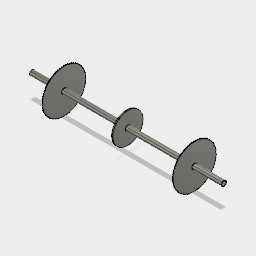
torsional analysis (Autodesk Fusion 360 design; units mm, degrees)
Autodesk Fusion 360 part; units mm, degrees
note: some values were not read from the file. Chosen so that the rebuilt part matches the saved one: which face or edge a step refers to; that a step has no effect.
sketch "Sketch1" plane through (0, 0, 0) normal (0, 0, 1) x (1, 0, 0)
  line L0 (0, 0) -> (-914.4, 0)
  dimension "d1" = 914.4
  measures "d1" distance of L0.start L0.end
pipe "Pipe1" add diameter 25.4 wall 2 path "Sketch1" along L0
ref_plane "WorkPlane1" through (-140, 0, 0) normal (1, 0, 0) x (0, 0, -1)
sketch "Sketch2" plane through (-140, 0, 0) normal (1, 0, 0) x (0, 0, -1)
  line L0 (-0.0125, 104.6) -> (0.9875, 104.6)
  line L1 (-0.0125, 104.6) -> (-1.0125, 104.6)
  line L2 (-9.8073, 104.1392) -> (-8.8117, 104.2329)
  line L3 (-9.8073, 104.1392) -> (-10.8029, 104.0456)
  line L4 (-19.516, 102.7633) -> (-18.5335, 102.9497)
  line L5 (-19.516, 102.7633) -> (-20.4984, 102.5768)
  line L6 (-29.0531, 100.4842) -> (-28.0924, 100.7619)
  line L7 (-29.0531, 100.4842) -> (-30.0138, 100.2066)
  line L8 (-38.3349, 97.3221) -> (-37.4045, 97.6885)
  line L9 (-38.3349, 97.3221) -> (-39.2654, 96.9557)
  line L10 (-47.2799, 93.3047) -> (-46.3878, 93.7566)
  line L11 (-47.2799, 93.3047) -> (-48.172, 92.8528)
  line L12 (-55.8093, 88.4674) -> (-54.9635, 89.0008)
  line L13 (-55.8093, 88.4674) -> (-56.6552, 87.9339)
  line L14 (-63.8483, 82.8526) -> (-63.0562, 83.4629)
  line L15 (-63.8483, 82.8526) -> (-64.6405, 82.2423)
  line L16 (-71.3262, 76.5097) -> (-70.5947, 77.1915)
  line L17 (-71.3262, 76.5097) -> (-72.0577, 75.8279)
  line L18 (-78.1773, 69.4944) -> (-77.5128, 70.2417)
  line L19 (-78.1773, 69.4944) -> (-78.8418, 68.7471)
  line L20 (-84.3413, 61.8684) -> (-83.7498, 62.6747)
  line L21 (-84.3413, 61.8684) -> (-84.9329, 61.0622)
  line L22 (-89.7642, 53.6987) -> (-89.2507, 54.5568)
  line L23 (-89.7642, 53.6987) -> (-90.2777, 52.8406)
  line L24 (-94.3982, 45.0571) -> (-93.9673, 45.9595)
  line L25 (-94.3982, 45.0571) -> (-94.829, 44.1547)
  line L26 (-98.2026, 36.0195) -> (-97.8581, 36.9583)
  line L27 (-98.2026, 36.0195) -> (-98.5471, 35.0807)
  line L28 (-101.144, 26.6654) -> (-100.889, 27.6324)
  line L29 (-101.144, 26.6654) -> (-101.3991, 25.6985)
  line L30 (-103.1966, 17.077) -> (-103.0332, 18.0635)
  line L31 (-103.1966, 17.077) -> (-103.36, 16.0904)
  line L32 (-104.3423, 7.3385) -> (-104.272, 8.336)
  line L33 (-104.3423, 7.3385) -> (-104.4125, 6.3409)
  line L34 (-104.571, -2.4645) -> (-104.5944, -1.4648)
  line L35 (-104.571, -2.4645) -> (-104.5475, -3.4643)
  line L36 (-103.8807, -12.2459) -> (-103.9976, -11.2528)
  line L37 (-103.8807, -12.2459) -> (-103.7637, -13.239)
  line L38 (-102.2775, -21.9196) -> (-102.487, -20.9418)
  line L39 (-102.2775, -21.9196) -> (-102.0681, -22.8975)
  line L40 (-99.7755, -31.4007) -> (-100.0756, -30.4468)
  line L41 (-99.7755, -31.4007) -> (-99.4754, -32.3546)
  line L42 (-96.3967, -40.6059) -> (-96.7848, -39.6843)
  line L43 (-96.3967, -40.6059) -> (-96.0086, -41.5275)
  line L44 (-92.1707, -49.4542) -> (-92.6434, -48.573)
  line L45 (-92.1707, -49.4542) -> (-91.698, -50.3354)
  line L46 (-87.1348, -57.8679) -> (-87.6879, -57.0348)
  line L47 (-87.1348, -57.8679) -> (-86.5816, -58.701)
  line L48 (-81.3331, -65.7731) -> (-81.9618, -64.9954)
  line L49 (-81.3331, -65.7731) -> (-80.7043, -66.5507)
  line L50 (-74.8166, -73.1002) -> (-75.5154, -72.3848)
  line L51 (-74.8166, -73.1002) -> (-74.1178, -73.8155)
  line L52 (-67.6426, -79.7849) -> (-68.4053, -79.1382)
  line L53 (-67.6426, -79.7849) -> (-66.8799, -80.4317)
  line L54 (-59.8742, -85.7685) -> (-60.6941, -85.196)
  line L55 (-59.8742, -85.7685) -> (-59.0543, -86.341)
  line L56 (-51.5797, -90.9983) -> (-52.4496, -90.5051)
  line L57 (-51.5797, -90.9983) -> (-50.7097, -91.4916)
  line L58 (-42.8318, -95.4285) -> (-43.7441, -95.0189)
  line L59 (-42.8318, -95.4285) -> (-41.9195, -95.8381)
  line L60 (-33.7075, -99.02) -> (-34.6541, -98.6976)
  line L61 (-33.7075, -99.02) -> (-32.7609, -99.3424)
  line L62 (-24.287, -101.7413) -> (-25.2597, -101.509)
  line L63 (-24.287, -101.7413) -> (-23.3144, -101.9736)
  line L64 (-14.6531, -103.5686) -> (-15.6432, -103.4284)
  line L65 (-14.6531, -103.5686) -> (-13.663, -103.7088)
  line L66 (-4.8904, -104.4856) -> (-5.8893, -104.4387)
  line L67 (-4.8904, -104.4856) -> (-3.8915, -104.5325)
  line L68 (4.9153, -104.4844) -> (3.9164, -104.5313)
  line L69 (4.9153, -104.4844) -> (5.9142, -104.4376)
  line L70 (14.6778, -103.5651) -> (13.6876, -103.7053)
  line L71 (14.6778, -103.5651) -> (15.6679, -103.4249)
  line L72 (24.3113, -101.7356) -> (23.3386, -101.9679)
  line L73 (24.3113, -101.7356) -> (25.2839, -101.5032)
  line L74 (33.7311, -99.012) -> (32.7845, -99.3343)
  line L75 (33.7311, -99.012) -> (34.6777, -98.6896)
  line L76 (42.8545, -95.4183) -> (41.9422, -95.8279)
  line L77 (42.8545, -95.4183) -> (43.7668, -95.0087)
  line L78 (51.6013, -90.9861) -> (50.7314, -91.4793)
  line L79 (51.6013, -90.9861) -> (52.4712, -90.4928)
  line L80 (59.8947, -85.7542) -> (59.0748, -86.3268)
  line L81 (59.8947, -85.7542) -> (60.7146, -85.1817)
  line L82 (67.6616, -79.7688) -> (66.8989, -80.4156)
  line L83 (67.6616, -79.7688) -> (68.4243, -79.122)
  line L84 (74.834, -73.0824) -> (74.1352, -73.7977)
  line L85 (74.834, -73.0824) -> (75.5328, -72.367)
  line L86 (81.3487, -65.7537) -> (80.72, -66.5313)
  line L87 (81.3487, -65.7537) -> (81.9774, -64.976)
  line L88 (87.1485, -57.8471) -> (86.5954, -58.6802)
  line L89 (87.1485, -57.8471) -> (87.7017, -57.014)
  line L90 (92.1825, -49.4322) -> (91.7098, -50.3135)
  line L91 (92.1825, -49.4322) -> (92.6552, -48.551)
  line L92 (96.4064, -40.5829) -> (96.0183, -41.5045)
  line L93 (96.4064, -40.5829) -> (96.7944, -39.6613)
  line L94 (99.783, -31.377) -> (99.4829, -32.3309)
  line L95 (99.783, -31.377) -> (100.0831, -30.4231)
  line L96 (102.2827, -21.8953) -> (102.0733, -22.8731)
  line L97 (102.2827, -21.8953) -> (102.4922, -20.9175)
  line L98 (103.8836, -12.2212) -> (103.7666, -13.2143)
  line L99 (103.8836, -12.2212) -> (104.0006, -11.228)
  line L100 (104.5715, -2.4396) -> (104.5481, -3.4394)
  line L101 (104.5715, -2.4396) -> (104.595, -1.4399)
  line L102 (104.3405, 7.3633) -> (104.4108, 6.3658)
  line L103 (104.3405, 7.3633) -> (104.2702, 8.3608)
  line L104 (103.1925, 17.1016) -> (103.3559, 16.115)
  line L105 (103.1925, 17.1016) -> (103.0291, 18.0881)
  line L106 (101.1377, 26.6895) -> (101.3927, 25.7226)
  line L107 (101.1377, 26.6895) -> (100.8826, 27.6564)
  line L108 (98.194, 36.0429) -> (98.5385, 35.1041)
  line L109 (98.194, 36.0429) -> (97.8496, 36.9817)
  line L110 (94.3875, 45.0796) -> (94.8183, 44.1772)
  line L111 (94.3875, 45.0796) -> (93.9566, 45.982)
  line L112 (89.7514, 53.7201) -> (90.2649, 52.862)
  line L113 (89.7514, 53.7201) -> (89.2379, 54.5782)
  line L114 (84.3266, 61.8885) -> (84.9182, 61.0822)
  line L115 (84.3266, 61.8885) -> (83.735, 62.6947)
  line L116 (78.1607, 69.513) -> (78.8252, 68.7657)
  line L117 (78.1607, 69.513) -> (77.4963, 70.2603)
  line L118 (71.308, 76.5267) -> (72.0395, 75.8449)
  line L119 (71.308, 76.5267) -> (70.5765, 77.2085)
  line L120 (63.8286, 82.8678) -> (64.6207, 82.2575)
  line L121 (63.8286, 82.8678) -> (63.0364, 83.4781)
  line L122 (55.7883, 88.4807) -> (56.6341, 87.9472)
  line L123 (55.7883, 88.4807) -> (54.9424, 89.0141)
  line L124 (47.2577, 93.316) -> (48.1497, 92.8641)
  line L125 (47.2577, 93.316) -> (46.3656, 93.7679)
  line L126 (38.3118, 97.3312) -> (39.2422, 96.9649)
  line L127 (38.3118, 97.3312) -> (37.3813, 97.6976)
  line L128 (29.0292, 100.4911) -> (29.9899, 100.2135)
  line L129 (29.0292, 100.4911) -> (28.0685, 100.7688)
  line L130 (19.4915, 102.7679) -> (20.4739, 102.5814)
  line L131 (19.4915, 102.7679) -> (18.509, 102.9544)
  line L132 (9.7825, 104.1416) -> (10.7781, 104.0479)
  line L133 (9.7825, 104.1416) -> (8.7869, 104.2352)
  arc A0 (0.9875, 104.6) -> (8.7869, 104.2352) centre (4.9379, 105.5011) ccw
  arc A1 (-8.8117, 104.2329) -> (-1.0125, 104.6) centre (-4.9631, 105.4999) ccw
  arc A2 (-18.5335, 102.9497) -> (-10.8029, 104.0456) centre (-14.8204, 104.5716) ccw
  arc A3 (-28.0924, 100.7619) -> (-20.4984, 102.5768) centre (-24.5476, 102.7243) ccw
  arc A4 (-37.4045, 97.6885) -> (-30.0138, 100.2066) centre (-34.0589, 99.9742) ccw
  arc A5 (-46.3878, 93.7566) -> (-39.2654, 96.9557) centre (-43.271, 96.3456) ccw
  arc A6 (-54.9635, 89.0008) -> (-48.172, 92.8528) centre (-52.1028, 91.8703) ccw
  arc A7 (-63.0562, 83.4629) -> (-56.6552, 87.9339) centre (-60.4768, 86.5876) ccw
  arc A8 (-70.5947, 77.1915) -> (-64.6405, 82.2423) centre (-68.3192, 80.544) ccw
  arc A9 (-77.5128, 70.2417) -> (-72.0577, 75.8279) centre (-75.5613, 73.7926) ccw
  arc A10 (-83.7498, 62.6747) -> (-78.8418, 68.7471) centre (-82.1393, 66.3927) ccw
  arc A11 (-89.2507, 54.5568) -> (-84.9329, 61.0622) centre (-87.9955, 58.4093) ccw
  arc A12 (-93.9673, 45.9595) -> (-90.2777, 52.8406) centre (-93.0784, 49.9126) ccw
  arc A13 (-97.8581, 36.9583) -> (-94.829, 44.1547) centre (-97.3433, 40.9773) ccw
  arc A14 (-100.889, 27.6324) -> (-98.5471, 35.0807) centre (-100.7528, 31.6819) ccw
  arc A15 (-103.0332, 18.0635) -> (-101.3991, 25.6985) centre (-103.2768, 22.108) ccw
  arc A16 (-104.272, 8.336) -> (-103.36, 16.0904) centre (-104.8932, 12.3399) ccw
  arc A17 (-104.5944, -1.4648) -> (-104.4125, 6.3409) centre (-105.5878, 2.4633) ccw
  arc A18 (-103.9976, -11.2528) -> (-104.5475, -3.4643) centre (-105.3546, -7.4349) ccw
  arc A19 (-102.487, -20.9418) -> (-103.7637, -13.239) centre (-104.1954, -17.2678) ccw
  arc A20 (-100.0756, -30.4468) -> (-102.0681, -22.8975) centre (-102.1206, -26.9489) ccw
  arc A21 (-96.7848, -39.6843) -> (-99.4754, -32.3546) centre (-99.1483, -36.3932) ccw
  arc A22 (-92.6434, -48.573) -> (-96.0086, -41.5275) centre (-95.3048, -45.5177) ccw
  arc A23 (-87.6879, -57.0348) -> (-91.698, -50.3354) centre (-90.6236, -54.2422) ccw
  arc A24 (-81.9618, -64.9954) -> (-86.5816, -58.701) centre (-85.1461, -62.49) ccw
  arc A25 (-75.5154, -72.3848) -> (-80.7043, -66.5507) centre (-78.9203, -70.1886) ccw
  arc A26 (-68.4053, -79.1382) -> (-74.1178, -73.8155) centre (-72.001, -77.2704) ccw
  arc A27 (-60.6941, -85.196) -> (-66.8799, -80.4317) centre (-64.4489, -83.6732) ccw
  arc A28 (-52.4496, -90.5051) -> (-59.0543, -86.341) centre (-56.3304, -89.3406) ccw
  arc A29 (-43.7441, -95.0189) -> (-50.7097, -91.4916) centre (-47.7169, -94.2229) ccw
  arc A30 (-34.6541, -98.6976) -> (-41.9195, -95.8381) centre (-38.6841, -98.2772) ccw
  arc A31 (-25.2597, -101.509) -> (-32.7609, -99.3424) centre (-29.3113, -101.4678) ccw
  arc A32 (-15.6432, -103.4284) -> (-23.3144, -101.9736) centre (-19.6809, -103.7667) ccw
  arc A33 (-5.8893, -104.4387) -> (-13.663, -103.7088) centre (-9.8775, -105.1537) ccw
  arc A34 (3.9164, -104.5313) -> (-3.8915, -104.5325) centre (0.0126, -105.6166) ccw
  arc A35 (13.6876, -103.7053) -> (5.9142, -104.4376) centre (9.9026, -105.1513) ccw
  arc A36 (23.3386, -101.9679) -> (15.6679, -103.4249) centre (19.7057, -103.762) ccw
  arc A37 (32.7845, -99.3343) -> (25.2839, -101.5032) centre (29.3355, -101.4608) ccw
  arc A38 (41.9422, -95.8279) -> (34.6777, -98.6896) centre (38.7075, -98.2679) ccw
  arc A39 (50.7314, -91.4793) -> (43.7668, -95.0087) centre (47.7394, -94.2115) ccw
  arc A40 (59.0748, -86.3268) -> (52.4712, -90.4928) centre (56.3517, -89.3272) ccw
  arc A41 (66.8989, -80.4156) -> (60.7146, -85.1817) centre (64.4689, -83.6578) ccw
  arc A42 (74.1352, -73.7977) -> (68.4243, -79.122) centre (72.0194, -77.2532) ccw
  arc A43 (80.72, -66.5313) -> (75.5328, -72.367) centre (78.9371, -70.1698) ccw
  arc A44 (86.5954, -58.6802) -> (81.9774, -64.976) centre (85.161, -62.4697) ccw
  arc A45 (91.7098, -50.3135) -> (87.7017, -57.014) centre (90.6366, -54.2206) ccw
  arc A46 (96.0183, -41.5045) -> (92.6552, -48.551) centre (95.3156, -45.495) ccw
  arc A47 (99.4829, -32.3309) -> (96.7944, -39.6613) centre (99.157, -36.3696) ccw
  arc A48 (102.0733, -22.8731) -> (100.0831, -30.4231) centre (102.127, -26.9246) ccw
  arc A49 (103.7666, -13.2143) -> (102.4922, -20.9175) centre (104.1995, -17.2429) ccw
  arc A50 (104.5481, -3.4394) -> (104.0006, -11.228) centre (105.3563, -7.4098) ccw
  arc A51 (104.4108, 6.3658) -> (104.595, -1.4399) centre (105.5872, 2.4885) ccw
  arc A52 (103.3559, 16.115) -> (104.2702, 8.3608) centre (104.8903, 12.3649) ccw
  arc A53 (101.3927, 25.7226) -> (103.0291, 18.0881) centre (103.2715, 22.1327) ccw
  arc A54 (98.5385, 35.1041) -> (100.8826, 27.6564) centre (100.7452, 31.7059) ccw
  arc A55 (94.8183, 44.1772) -> (97.8496, 36.9817) centre (97.3335, 41.0005) ccw
  arc A56 (90.2649, 52.862) -> (93.9566, 45.982) centre (93.0665, 49.9348) ccw
  arc A57 (84.9182, 61.0822) -> (89.2379, 54.5782) centre (87.9816, 58.4303) ccw
  arc A58 (78.8252, 68.7657) -> (83.735, 62.6947) centre (82.1235, 66.4123) ccw
  arc A59 (72.0395, 75.8449) -> (77.4963, 70.2603) centre (75.5437, 73.8106) ccw
  arc A60 (64.6207, 82.2575) -> (70.5765, 77.2085) centre (68.3, 80.5603) ccw
  arc A61 (56.6341, 87.9472) -> (63.0364, 83.4781) centre (60.4561, 86.6021) ccw
  arc A62 (48.1497, 92.8641) -> (54.9424, 89.0141) centre (52.0809, 91.8827) ccw
  arc A63 (39.2422, 96.9649) -> (46.3656, 93.7679) centre (43.248, 96.3559) ccw
  arc A64 (29.9899, 100.2135) -> (37.3813, 97.6976) centre (34.0351, 99.9824) ccw
  arc A65 (20.4739, 102.5814) -> (28.0685, 100.7688) centre (24.523, 102.7301) ccw
  arc A66 (10.7781, 104.0479) -> (18.509, 102.9544) centre (14.7955, 104.5751) ccw
  dimension "d9" = 1
  dimension "d10" = 1
  dimension "d12" = 360
  dimension "d14" = 360
  measures "d9" distance of L0.start L0.end
  measures "d10" distance of L0.start L1.end
ref_plane "WorkPlane3" through (-764.4, 0, 0) normal (-1, 0, 0) x (0, 0, 1)
sketch "Sketch3" plane through (-764.4, 0, 0) normal (-1, 0, 0) x (0, 0, -1)
  line L0 (-0.0279, -104.6) -> (0.9721, -104.6)
  line L1 (-0.0279, -104.6) -> (-1.0279, -104.6)
  line L2 (9.7672, -104.143) -> (8.7716, -104.2366)
  line L3 (9.7672, -104.143) -> (10.7628, -104.0494)
  line L4 (19.4764, -102.7708) -> (18.4939, -102.9572)
  line L5 (19.4764, -102.7708) -> (20.4588, -102.5843)
  line L6 (29.0144, -100.4954) -> (28.0537, -100.773)
  line L7 (29.0144, -100.4954) -> (29.9751, -100.2178)
  line L8 (38.2974, -97.3369) -> (37.367, -97.7033)
  line L9 (38.2974, -97.3369) -> (39.2279, -96.9705)
  line L10 (47.2439, -93.3229) -> (46.3519, -93.7748)
  line L11 (47.2439, -93.3229) -> (48.136, -92.871)
  line L12 (55.7752, -88.4889) -> (54.9294, -89.0223)
  line L13 (55.7752, -88.4889) -> (56.6211, -87.9554)
  line L14 (63.8164, -82.8772) -> (63.0242, -83.4875)
  line L15 (63.8164, -82.8772) -> (64.6086, -82.2669)
  line L16 (71.2967, -76.5372) -> (70.5652, -77.219)
  line L17 (71.2967, -76.5372) -> (72.0283, -75.8554)
  line L18 (78.1505, -69.5245) -> (77.486, -70.2718)
  line L19 (78.1505, -69.5245) -> (78.815, -68.7772)
  line L20 (84.3175, -61.9009) -> (83.7259, -62.7072)
  line L21 (84.3175, -61.9009) -> (84.9091, -61.0947)
  line L22 (89.7435, -53.7333) -> (89.23, -54.5914)
  line L23 (89.7435, -53.7333) -> (90.257, -52.8752)
  line L24 (94.3808, -45.0935) -> (93.95, -45.9959)
  line L25 (94.3808, -45.0935) -> (94.8117, -44.1911)
  line L26 (98.1887, -36.0574) -> (97.8443, -36.9962)
  line L27 (98.1887, -36.0574) -> (98.5332, -35.1186)
  line L28 (101.1337, -26.7044) -> (100.8787, -27.6713)
  line L29 (101.1337, -26.7044) -> (101.3888, -25.7375)
  line L30 (103.19, -17.1168) -> (103.0266, -18.1033)
  line L31 (103.19, -17.1168) -> (103.3534, -16.1302)
  line L32 (104.3394, -7.3787) -> (104.2691, -8.3762)
  line L33 (104.3394, -7.3787) -> (104.4097, -6.3811)
  line L34 (104.5719, 2.4242) -> (104.5953, 1.4245)
  line L35 (104.5719, 2.4242) -> (104.5485, 3.424)
  line L36 (103.8854, 12.2059) -> (104.0024, 11.2127)
  line L37 (103.8854, 12.2059) -> (103.7684, 13.199)
  line L38 (102.286, 21.8802) -> (102.4954, 20.9024)
  line L39 (102.286, 21.8802) -> (102.0765, 22.858)
  line L40 (99.7876, 31.3623) -> (100.0877, 30.4084)
  line L41 (99.7876, 31.3623) -> (99.4875, 32.3162)
  line L42 (96.4123, 40.5687) -> (96.8004, 39.6471)
  line L43 (96.4123, 40.5687) -> (96.0242, 41.4904)
  line L44 (92.1898, 49.4187) -> (92.6625, 48.5374)
  line L45 (92.1898, 49.4187) -> (91.7171, 50.2999)
  line L46 (87.1571, 57.8343) -> (87.7102, 57.0012)
  line L47 (87.1571, 57.8343) -> (86.6039, 58.6674)
  line L48 (81.3584, 65.7417) -> (81.9871, 64.9641)
  line L49 (81.3584, 65.7417) -> (80.7297, 66.5193)
  line L50 (74.8448, 73.0714) -> (75.5435, 72.356)
  line L51 (74.8448, 73.0714) -> (74.146, 73.7867)
  line L52 (67.6734, 79.7589) -> (68.4361, 79.1121)
  line L53 (67.6734, 79.7589) -> (66.9107, 80.4056)
  line L54 (59.9073, 85.7454) -> (60.7272, 85.1729)
  line L55 (59.9073, 85.7454) -> (59.0874, 86.3179)
  line L56 (51.6147, 90.9785) -> (52.4846, 90.4852)
  line L57 (51.6147, 90.9785) -> (50.7448, 91.4717)
  line L58 (42.8686, 95.412) -> (43.7808, 95.0024)
  line L59 (42.8686, 95.412) -> (41.9563, 95.8216)
  line L60 (33.7457, 99.007) -> (34.6923, 98.6847)
  line L61 (33.7457, 99.007) -> (32.7991, 99.3294)
  line L62 (24.3262, 101.732) -> (25.2989, 101.4997)
  line L63 (24.3262, 101.732) -> (23.3536, 101.9643)
  line L64 (14.693, 103.5629) -> (15.6831, 103.4227)
  line L65 (14.693, 103.5629) -> (13.7029, 103.7031)
  line L66 (4.9307, 104.4837) -> (5.9296, 104.4369)
  line L67 (4.9307, 104.4837) -> (3.9318, 104.5306)
  line L68 (-4.875, 104.4863) -> (-3.8761, 104.5332)
  line L69 (-4.875, 104.4863) -> (-5.8739, 104.4395)
  line L70 (-14.6379, 103.5707) -> (-13.6477, 103.7109)
  line L71 (-14.6379, 103.5707) -> (-15.628, 103.4305)
  line L72 (-24.272, 101.7449) -> (-23.2994, 101.9772)
  line L73 (-24.272, 101.7449) -> (-25.2447, 101.5126)
  line L74 (-33.6929, 99.025) -> (-32.7463, 99.3473)
  line L75 (-33.6929, 99.025) -> (-34.6396, 98.7026)
  line L76 (-42.8177, 95.4348) -> (-41.9055, 95.8444)
  line L77 (-42.8177, 95.4348) -> (-43.73, 95.0252)
  line L78 (-51.5663, 91.0059) -> (-50.6963, 91.4992)
  line L79 (-51.5663, 91.0059) -> (-52.4362, 90.5127)
  line L80 (-59.8616, 85.7773) -> (-59.0417, 86.3498)
  line L81 (-59.8616, 85.7773) -> (-60.6815, 85.2048)
  line L82 (-67.6309, 79.7949) -> (-66.8682, 80.4417)
  line L83 (-67.6309, 79.7949) -> (-68.3936, 79.1481)
  line L84 (-74.8058, 73.1112) -> (-74.1071, 73.8266)
  line L85 (-74.8058, 73.1112) -> (-75.5046, 72.3959)
  line L86 (-81.3234, 65.785) -> (-80.6947, 66.5627)
  line L87 (-81.3234, 65.785) -> (-81.9521, 65.0074)
  line L88 (-87.1262, 57.8807) -> (-86.5731, 58.7138)
  line L89 (-87.1262, 57.8807) -> (-87.6794, 57.0476)
  line L90 (-92.1634, 49.4678) -> (-91.6908, 50.349)
  line L91 (-92.1634, 49.4678) -> (-92.6361, 48.5865)
  line L92 (-96.3907, 40.6201) -> (-96.0026, 41.5417)
  line L93 (-96.3907, 40.6201) -> (-96.7788, 39.6985)
  line L94 (-99.7709, 31.4154) -> (-99.4708, 32.3693)
  line L95 (-99.7709, 31.4154) -> (-100.071, 30.4615)
  line L96 (-102.2743, 21.9347) -> (-102.0648, 22.9125)
  line L97 (-102.2743, 21.9347) -> (-102.4837, 20.9569)
  line L98 (-103.8789, 12.2612) -> (-103.7619, 13.2543)
  line L99 (-103.8789, 12.2612) -> (-103.9958, 11.2681)
  line L100 (-104.5706, 2.4799) -> (-104.5472, 3.4797)
  line L101 (-104.5706, 2.4799) -> (-104.594, 1.4802)
  line L102 (-104.3433, -7.3231) -> (-104.4136, -6.3256)
  line L103 (-104.3433, -7.3231) -> (-104.2731, -8.3206)
  line L104 (-103.1991, -17.0618) -> (-103.3625, -16.0752)
  line L105 (-103.1991, -17.0618) -> (-103.0357, -18.0484)
  line L106 (-101.148, -26.6505) -> (-101.403, -25.6836)
  line L107 (-101.148, -26.6505) -> (-100.8929, -27.6175)
  line L108 (-98.2079, -36.0051) -> (-98.5524, -35.0663)
  line L109 (-98.2079, -36.0051) -> (-97.8634, -36.9439)
  line L110 (-94.4048, -45.0432) -> (-94.8357, -44.1408)
  line L111 (-94.4048, -45.0432) -> (-93.974, -45.9456)
  line L112 (-89.7721, -53.6855) -> (-90.2856, -52.8274)
  line L113 (-89.7721, -53.6855) -> (-89.2586, -54.5436)
  line L114 (-84.3504, -61.856) -> (-84.942, -61.0497)
  line L115 (-84.3504, -61.856) -> (-83.7589, -62.6622)
  line L116 (-78.1875, -69.4829) -> (-78.852, -68.7356)
  line L117 (-78.1875, -69.4829) -> (-77.523, -70.2302)
  line L118 (-71.3375, -76.4992) -> (-72.069, -75.8174)
  line L119 (-71.3375, -76.4992) -> (-70.6059, -77.181)
  line L120 (-63.8605, -82.8432) -> (-64.6527, -82.2329)
  line L121 (-63.8605, -82.8432) -> (-63.0684, -83.4535)
  line L122 (-55.8224, -88.4592) -> (-56.6682, -87.9257)
  line L123 (-55.8224, -88.4592) -> (-54.9765, -88.9926)
  line L124 (-47.2936, -93.2978) -> (-48.1857, -92.8459)
  line L125 (-47.2936, -93.2978) -> (-46.4016, -93.7497)
  line L126 (-38.3493, -97.3165) -> (-39.2797, -96.9501)
  line L127 (-38.3493, -97.3165) -> (-37.4188, -97.6828)
  line L128 (-29.0679, -100.4799) -> (-30.0286, -100.2023)
  line L129 (-29.0679, -100.4799) -> (-28.1072, -100.7576)
  line L130 (-19.5311, -102.7604) -> (-20.5135, -102.5739)
  line L131 (-19.5311, -102.7604) -> (-18.5486, -102.9468)
  line L132 (-9.8226, -104.1378) -> (-10.8182, -104.0441)
  line L133 (-9.8226, -104.1378) -> (-8.827, -104.2314)
  arc A0 (8.7716, -104.2366) -> (0.9721, -104.6) centre (4.9222, -105.499) ccw
  arc A1 (18.4939, -102.9572) -> (10.7628, -104.0494) centre (14.7797, -104.5745) ccw
  arc A2 (28.0537, -100.773) -> (20.4588, -102.5843) centre (24.5072, -102.731) ccw
  arc A3 (37.367, -97.7033) -> (29.9751, -100.2178) centre (34.0194, -99.9847) ccw
  arc A4 (46.3519, -93.7748) -> (39.2279, -96.9705) centre (43.2327, -96.3598) ccw
  arc A5 (54.9294, -89.0223) -> (48.136, -92.871) centre (52.066, -91.888) ccw
  arc A6 (63.0242, -83.4875) -> (56.6211, -87.9554) centre (60.4417, -86.6087) ccw
  arc A7 (70.5652, -77.219) -> (64.6086, -82.2669) centre (68.2863, -80.5683) ccw
  arc A8 (77.486, -70.2718) -> (72.0283, -75.8554) centre (75.5308, -73.8198) ccw
  arc A9 (83.7259, -62.7072) -> (78.815, -68.7772) centre (82.1115, -66.4226) ccw
  arc A10 (89.23, -54.5914) -> (84.9091, -61.0947) centre (87.9706, -58.4417) ccw
  arc A11 (93.95, -45.9959) -> (90.257, -52.8752) centre (93.0566, -49.9472) ccw
  arc A12 (97.8443, -36.9962) -> (94.8117, -44.1911) centre (97.3249, -41.0138) ccw
  arc A13 (100.8787, -27.6713) -> (98.5332, -35.1186) centre (100.7378, -31.7199) ccw
  arc A14 (103.0266, -18.1033) -> (101.3888, -25.7375) centre (103.2655, -22.1473) ccw
  arc A15 (104.2691, -8.3762) -> (103.3534, -16.1302) centre (104.8856, -12.3801) ccw
  arc A16 (104.5953, 1.4245) -> (104.4097, -6.3811) centre (105.5841, -2.504) ccw
  arc A17 (104.0024, 11.2127) -> (104.5485, 3.424) centre (105.3546, 7.394) ccw
  arc A18 (102.4954, 20.9024) -> (103.7684, 13.199) centre (104.1993, 17.2271) ccw
  arc A19 (100.0877, 30.4084) -> (102.0765, 22.858) centre (102.1283, 26.9088) ccw
  arc A20 (96.8004, 39.6471) -> (99.4875, 32.3162) centre (99.1597, 36.354) ccw
  arc A21 (92.6625, 48.5374) -> (96.0242, 41.4904) centre (95.3198, 45.4797) ccw
  arc A22 (87.7102, 57.0012) -> (91.7171, 50.2999) centre (90.6422, 54.2057) ccw
  arc A23 (81.9871, 64.9641) -> (86.6039, 58.6674) centre (85.168, 62.4554) ccw
  arc A24 (75.5435, 72.356) -> (80.7297, 66.5193) centre (78.9453, 70.1563) ccw
  arc A25 (68.4361, 79.1121) -> (74.146, 73.7867) centre (72.0289, 77.2406) ccw
  arc A26 (60.7272, 85.1729) -> (66.9107, 80.4056) centre (64.4795, 83.646) ccw
  arc A27 (52.4846, 90.4852) -> (59.0874, 86.3179) centre (56.3634, 89.3165) ccw
  arc A28 (43.7808, 95.0024) -> (50.7448, 91.4717) centre (47.752, 94.202) ccw
  arc A29 (34.6923, 98.6847) -> (41.9563, 95.8216) centre (38.721, 98.2596) ccw
  arc A30 (25.2989, 101.4997) -> (32.7991, 99.3294) centre (29.3497, 101.4537) ccw
  arc A31 (15.6831, 103.4227) -> (23.3536, 101.9643) centre (19.7204, 103.7563) ccw
  arc A32 (5.9296, 104.4369) -> (13.7029, 103.7031) centre (9.9179, 105.147) ccw
  arc A33 (-3.8761, 104.5332) -> (3.9318, 104.5306) centre (0.0282, 105.6137) ccw
  arc A34 (-13.6477, 103.7109) -> (-5.8739, 104.4395) centre (-9.8618, 105.1523) ccw
  arc A35 (-23.2994, 101.9772) -> (-15.628, 103.4305) centre (-19.6651, 103.7668) ccw
  arc A36 (-32.7463, 99.3473) -> (-25.2447, 101.5126) centre (-29.2955, 101.4694) ccw
  arc A37 (-41.9055, 95.8444) -> (-34.6396, 98.7026) centre (-38.6685, 98.2803) ccw
  arc A38 (-50.6963, 91.4992) -> (-43.73, 95.0252) centre (-47.7017, 94.2274) ccw
  arc A39 (-59.0417, 86.3498) -> (-52.4362, 90.5127) centre (-56.3157, 89.3465) ccw
  arc A40 (-66.8682, 80.4417) -> (-60.6815, 85.2048) centre (-64.4348, 83.6804) ccw
  arc A41 (-74.1071, 73.8266) -> (-68.3936, 79.1481) centre (-71.9877, 77.279) ccw
  arc A42 (-80.6947, 66.5627) -> (-75.5046, 72.3959) centre (-78.9079, 70.1984) ccw
  arc A43 (-86.5731, 58.7138) -> (-81.9521, 65.0074) centre (-85.1346, 62.5009) ccw
  arc A44 (-91.6908, 50.349) -> (-87.6794, 57.0476) centre (-90.6132, 54.2541) ccw
  arc A45 (-96.0026, 41.5417) -> (-92.6361, 48.5865) centre (-95.2955, 45.5306) ccw
  arc A46 (-99.4708, 32.3693) -> (-96.7788, 39.6985) centre (-99.1403, 36.4069) ccw
  arc A47 (-102.0648, 22.9125) -> (-100.071, 30.4615) centre (-102.1139, 26.9633) ccw
  arc A48 (-103.7619, 13.2543) -> (-102.4837, 20.9569) centre (-104.1901, 17.2827) ccw
  arc A49 (-104.5472, 3.4797) -> (-103.9958, 11.2681) centre (-105.3506, 7.4502) ccw
  arc A50 (-104.4136, -6.3256) -> (-104.594, 1.4802) centre (-105.5854, -2.4477) ccw
  arc A51 (-103.3625, -16.0752) -> (-104.2731, -8.3206) centre (-104.8922, -12.3241) ccw
  arc A52 (-101.403, -25.6836) -> (-103.0357, -18.0484) centre (-103.2773, -22.0922) ccw
  arc A53 (-98.5524, -35.0663) -> (-100.8929, -27.6175) centre (-100.7547, -31.6662) ccw
  arc A54 (-94.8357, -44.1408) -> (-97.8634, -36.9439) centre (-97.3468, -40.9619) ccw
  arc A55 (-90.2856, -52.8274) -> (-93.974, -45.9456) centre (-93.0833, -49.8976) ccw
  arc A56 (-84.942, -61.0497) -> (-89.2586, -54.5436) centre (-88.0018, -58.3948) ccw
  arc A57 (-78.852, -68.7356) -> (-83.7589, -62.6622) centre (-82.1469, -66.3788) ccw
  arc A58 (-72.069, -75.8174) -> (-77.523, -70.2302) centre (-75.5702, -73.7795) ccw
  arc A59 (-64.6527, -82.2329) -> (-70.6059, -77.181) centre (-68.3293, -80.5318) ccw
  arc A60 (-56.6682, -87.9257) -> (-63.0684, -83.4535) centre (-60.4879, -86.5764) ccw
  arc A61 (-48.1857, -92.8459) -> (-54.9765, -88.9926) centre (-52.115, -91.8602) ccw
  arc A62 (-39.2797, -96.9501) -> (-46.4016, -93.7497) centre (-43.2841, -96.3367) ccw
  arc A63 (-30.0286, -100.2023) -> (-37.4188, -97.6828) centre (-34.0728, -99.9665) ccw
  arc A64 (-20.5135, -102.5739) -> (-28.1072, -100.7576) centre (-24.5621, -102.7179) ccw
  arc A65 (-10.8182, -104.0441) -> (-18.5486, -102.9468) centre (-14.8355, -104.5666) ccw
  arc A66 (-1.0279, -104.6) -> (-8.827, -104.2314) centre (-4.9785, -105.4963) ccw
  dimension "d18" = 1
  dimension "d19" = 1
  dimension "d21" = 360
  dimension "d23" = 360
  measures "d18" distance of L0.start L0.end
  measures "d19" distance of L0.start L1.end
extrude "Extrude1" add sketch "Sketch3" against normal blind 3
extrude "Extrude2" add sketch "Sketch2" against normal blind 3
ref_plane "WorkPlane4" through (-457.2, 0, 0) normal (1, 0, 0) x (0, 0, -1)
sketch "Sketch4" plane through (-457.2, 0, 0) normal (1, 0, 0) x (0, 0, -1)
  circle A0 centre (0, 0) radius 72.6626
extrude "Extrude3" add sketch "Sketch4" against normal blind 6
split_face "SplitFace1" [no effect]
equation "d1 = ( 36 * 25.4 ) * 1 mm"
equation "d28 = -18 * 25.4 mm"
